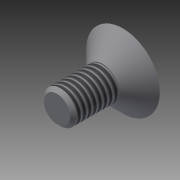
# Autodesk Inventor part: M5x10FHS
Saved by Autodesk Inventor 2015 (Build 190159000, 159)
## iProperties
Company: Misumi
Created: 2013-12-14
Part Number: M5x10FHS
Material: Generic
Document SubType Name: Modeling
Designer: Jack
Density: 1 g/cm^3
Appearance: Default
Author: Jack
Autodesk Inventor part; units mm, degrees
ref_plane "YZ Plane" through (0, 0, 0) normal (1, 0, 0) x (0, 1, 0)
ref_plane "XZ Plane" through (0, 0, 0) normal (0, 1, 0) x (-1, 0, 0)
ref_plane "XY Plane" through (0, 0, 0) normal (0, 0, 1) x (1, 0, 0)
sketch "Sketch1" plane through (0, 0, 0) normal (0, 1, 0) x (-1, 0, 0)
  circle A0 centre (0, 0) radius 5
  dimension "d0" = 10
  constraints: 1 centre point, 1 coincident
  measures "d0" diameter of A0
extrude "Extrusion1" add sketch "Sketch1" along normal blind 3.1
chamfer "Chamfer1" distance 3.1 angle 45 1 edges at (5, 0, 0)
sketch "Sketch2" plane through (0, 0, 0) normal (0, -1, 0) x (1, 0, 0)
  circle A0 centre (0, 0) radius 1.9 projected
  circle A1 centre (0, 0) radius 2.5
  dimension "d7" = 5
  constraints: 1 centre point, 1 coincident
  measures "d7" diameter of A1
extrude "Extrusion2" add sketch "Sketch2" along normal blind 6.9 and the other way blind 1 contours A0 | A1
chamfer "Chamfer2" distance 0.5 angle 45 1 edges at (-2.5, -6.9, 0)
sketch "Sketch3" plane through (0, 3.1, 0) normal (0, 1, 0) x (1, 0, 0)
  circle A0 centre (0, 0) radius 5 projected
  line L0 (0, 1.7321) -> (1.5, 0.866)
  line L1 (1.5, 0.866) -> (1.5, -0.866)
  line L2 (1.5, -0.866) -> (0, -1.7321)
  line L3 (0, -1.7321) -> (-1.5, -0.866)
  line L4 (-1.5, -0.866) -> (-1.5, 0.866)
  line L5 (-1.5, 0.866) -> (0, 1.7321)
  dimension "d15" = 3
  constraints: 12 end point, 1 coincident, 1 vertical, 13 other
  measures "d15" distance between parallel lines of L1 L4
extrude "Extrusion3" cut sketch "Sketch3" against normal blind 2 contours L0 L1 L2 L3 L4 L5
thread "Thread1" size "M5x0.8" class "6g" standard "ANSI Metric M Profile" full length
body "Solid1"
